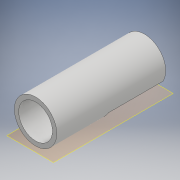
# Autodesk Inventor part: Motor sleeve
Saved by Autodesk Inventor 2017 (Build 210142000, 142)
## iProperties
Created: 2017-03-27
Part Number: Motor sleeve
Material: Generic
Document SubType Name: Modeling
Designer: yella
Density: 1 g/cm^3
Appearance: Default
Author: yella
Autodesk Inventor part; units mm, degrees
ref_plane "YZ Plane" through (0, 0, 0) normal (1, 0, 0) x (0, 1, 0)
ref_plane "XZ Plane" through (0, 0, 0) normal (0, 1, 0) x (-1, 0, 0)
sketch "Sketch1" plane through (0, 0, 0) normal (0, 1, 0) x (-1, 0, 0)
  circle A0 centre (0, 0) radius 1.55
  circle A1 centre (0, 0) radius 1.95
  dimension "d0" = 3.1
  dimension "d1" = 3.9
  constraints: 2 centre point, 2 coincident
  measures "d0" diameter of A0
  measures "d1" diameter of A1
extrude "Extrusion1" add sketch "Sketch1" along normal blind 10
ref_plane "Work Plane1" through (0, 0, -1.95) normal (0, 0, 1) x (1, 0, 0)
sketch "Sketch2" plane through (0, 0, -1.95) normal (0, 0, 1) x (1, 0, 0)
  line L0 (1.95, 10) -> (-1.95, 10) projected
  line L1 (-1.95, 10) -> (1.95, 10)
  line L2 (1.95, 10) -> (1.95, 5)
  line L3 (1.95, 5) -> (-1.95, 5)
  line L4 (-1.95, 5) -> (-1.95, 10)
  point P0 (0, 0)
  dimension "d4" = 5
  constraints: 8 end point, 2 parallel, 1 horizontal, 1 perpendicular
  measures "d4" distance of L0.start L2.end
extrude "Extrusion2" cut sketch "Sketch2" along normal blind 1
body "Solid1"
